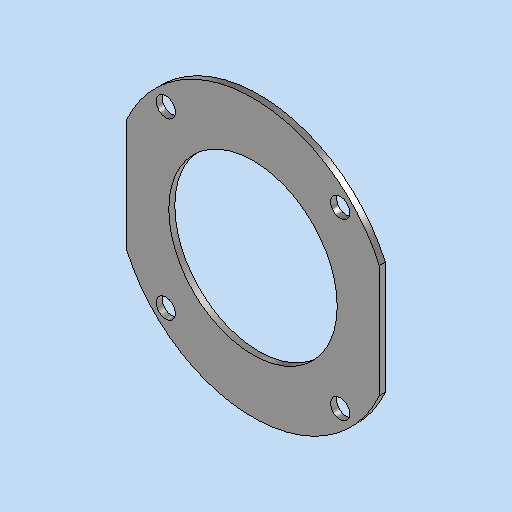
# Autodesk Inventor part: probe-gate-spacer-quartz-holder
Saved by Autodesk Inventor 2025 (Build 290162000, 162)
## iProperties
Created: 2024-05-15
Part Number: probe-gate-spacer-quartz-holder
Material: Stainless Steel
Document SubType Name: Modeling
Designer: queezz
Density: 8 g/cm^3
Appearance: Semi-Polished
Mass: 23.3231 g
Surface Area: 29.7529 cm^2
Volume: 2.91539 cm^3
Author: queezz
Autodesk Inventor part; units mm, degrees
ref_plane "YZ Plane" through (0, 0, 0) normal (1, 0, 0) x (0, 1, 0)
ref_plane "XZ Plane" through (0, 0, 0) normal (0, 1, 0) x (-1, 0, 0)
sketch "Sketch1" plane through (0, 0, 0) normal (0, 0, 1) x (1, 0, 0)
  circle A0 centre (0, 0) radius 14
  circle A1 centre (0, 0) radius 23
  dimension "d0" = 28
  dimension "d1" = 46
  constraints: 2 centre point, 2 coincident
  measures "d0" diameter of A0
  measures "d1" diameter of A1
extrude "Extrusion1" add sketch "Sketch1" along normal blind 10
sketch "Sketch2" plane through (0, 0, 10) normal (0, 0, 1) x (1, 0, 0)
  line L0 (0, 0) -> (23, 0) construction
  circle A0 centre (0, 0) radius 23 projected
  circle A1 centre (0, 0) radius 20.5 construction
  line L1 (0, 0) -> (14.4957, 14.4957) construction
  dimension "d35" = 41
  dimension "d34" = 45
  constraints: 4 end point, 2 coincident, 1 horizontal, 1 horizontal alignment, 4 other
  measures "d34" angle of L0 L1
hole "For-m3-screws" at (14.4957, 14.4957, 10) direction (0, 0, -1) diameter 3.2 end through all counterbore diameter 7 counterbore depth 8.5
fillet "Fillet3" radius 0.5 2 edges at (14.3283, 17.9917, 5.75) (17.9917, 14.3283, 5.75)
pattern_circular "Circular Pattern1" count 4 over 360 about axis through (0, 0, 0) along (0, 0, 1) of "For-m3-screws", "Fillet3"
sketch "Sketch3" plane through (0, 0, 0) normal (0, 1, 0) x (-1, 0, 0)
  line L0 (23, 3.8135) -> (-23, 1)
  line L1 (-23, 1) -> (-23, 11)
  line L2 (23, 10) -> (-27, 10) projected
  line L3 (-23, 11) -> (23, 11)
  line L4 (23, 11) -> (23, 3.8135)
  line L5 (-23, 0) -> (-23, 10) projected
  line L6 (23, 0) -> (23, 10) projected
  line L7 (-14, 0) -> (14, 0) projected
  line L8 (-27, 10) -> (-23, 10) projected
  point P0 (0, 0)
  point P1 (-14.3283, 10)
  point P2 (0, 11)
  point P3 (-17.9917, 10)
  dimension "d14" = 3.5
  dimension "d15" = 1
  dimension "d16" = 1
  constraints: 8 end point, 3 perpendicular, 1 midpoint, 1 point on line, 1 vertical alignment
  measures "d14" angle of L7 L0
  measures "d15" distance of L5.start L0.end
  measures "d16" distance between parallel lines of L3 L8
extrude "Angled-cut" [suppressed]
sketch "Sketch6" plane through (0, 0, 0) normal (0, 1, 0) x (-1, 0, 0)
  line L0 (23, 10) -> (-23, 10)
  line L1 (-23, 10) -> (-23, 1)
  line L2 (-23, 1) -> (23, 1)
  line L3 (23, 1) -> (23, 10)
  line L4 (23, 0) -> (-23, 0) projected
  line L5 (23, 0) -> (23, 10) projected
  line L6 (-23, 0) -> (-23, 10) projected
  point P0 (0, 0)
  point P1 (0, 10)
  dimension "d27" = 1
  constraints: 8 end point, 2 parallel, 1 horizontal, 1 midpoint, 1 perpendicular, 1 vertical alignment
  measures "d27" distance between parallel lines of L4 L2
extrude "Straight-cut" cut sketch "Sketch6" along normal through all both and the other way through all contours L3 L2 L1 L0
sketch "Sketch4" plane through (0, 0, 0) normal (0, 0, 1) x (1, 0, 0)
  line L0 (21, 30) -> (26, 30)
  line L1 (26, 30) -> (26, -30)
  line L2 (26, -30) -> (21, -30)
  line L3 (21, -30) -> (21, 30)
  point P0 (0, 0)
  point P1 (26, 0)
  dimension "d19" = 21
  dimension "d20" = 60
  dimension "d21" = 5
  constraints: 8 end point, 2 parallel, 1 horizontal, 1 horizontal alignment, 1 midpoint, 1 perpendicular
  measures "d19" distance from line of L3 point (0, 0)
  measures "d20" distance of L0.end L1.end
  measures "d21" distance of L0.start L0.end
extrude "Extrusion3" cut sketch "Sketch4" along normal blind 10
mirror "Mirror1" about plane through (0, 0, 0) normal (1, 0, 0) of "Extrusion3"
ref_plane "Work Plane1" through (22, -12.0416, 0) normal (1, 0, 0) x (0, 0, -1)
sketch "Sketch8" plane through (22, -12.0416, 0) normal (1, 0, 0) x (0, 0, -1)
  line L0 (-0.5, 21.0416) -> (-0.5, 3.0416) construction
  line L1 (-1, 2.6608) -> (-1, 21.4224) projected
  line L2 (0, 21.4224) -> (0, 2.6608) projected
  line L3 (0, 12.0416) -> (-1, 12.0416) construction
  point P0 (-0.5, 12.0416)
  dimension "d41" = 18
  constraints: 4 end point, 3 midpoint, 2 coincident, 1 horizontal alignment, 1 vertical
  measures "d41" distance of L0.start L0.end
hole "Hole2" [suppressed]
chamfer "Chamfer1" [suppressed]
thread "Thread2" size "M2x0.4" class "6H" standard "ANSI Metric M Profile" full length
thread "Thread3" size "M2x0.4" class "6H" standard "ANSI Metric M Profile" full length
thread "Thread4" size "M2x0.4" class "6H" standard "ANSI Metric M Profile" full length
thread "Thread5" size "M2x0.4" class "6H" standard "ANSI Metric M Profile" full length
equation "\"d0\" = innerdiameter"
equation "\"d1\" = outerdiameter"
equation "\"d35\" = holepositiondiameter"
equation "\"d19\" = trimspan"
equation "\"outerdiameter\" = 46"
equation "\"innerdiameter\" = 28"
equation "\"holepositiondiameter\" = 41"
equation "\"trimspan\" = 21"
body "Solid1"
